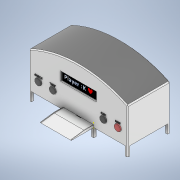
# Autodesk Inventor part: Twist Body
Saved by Autodesk Inventor 2021 (Build 250183000, 183)
## iProperties
Created: 2021-03-24
Part Number: Twist Body
Material: Generic
Document SubType Name: Modeling
Designer: calst
Density: 1 g/cm^3
Appearance: Smooth - White
Author: calst
Autodesk Inventor part; units mm, degrees
ref_plane "YZ Plane" through (0, 0, 0) normal (1, 0, 0) x (0, 1, 0)
ref_plane "XZ Plane" through (0, 0, 0) normal (0, 1, 0) x (-1, 0, 0)
sketch "Sketch1" plane through (0, 0, 0) normal (0, 1, 0) x (-1, 0, 0)
  line L0 (0, 0) -> (68.5, 0)
  line L1 (68.5, 0) -> (68.5, -94)
  line L2 (68.5, -94) -> (0, -94)
  line L3 (0, -94) -> (0, 0)
  dimension "d0" = 94
  dimension "d1" = 68.5
  constraints: 8 end point, 2 parallel, 1 horizontal, 1 perpendicular
  measures "d0" distance of L0.end L1.end
  measures "d1" distance of L1.end L2.end
extrude "Extrusion1" add sketch "Sketch1" along normal blind 4
sketch "Sketch2" plane through (0, 4, 0) normal (0, 1, 0) x (1, 0, 0)
  line L0 (0, 94) -> (-68.5, 94) projected
  line L1 (-68.5, 0) -> (0, 0) projected
  line L2 (-34.25, 0) -> (-39.25, 0)
  line L3 (-39.25, 0) -> (-39.25, 94)
  line L4 (-39.25, 94) -> (-29.25, 94)
  line L5 (-29.25, 94) -> (-29.25, 0)
  line L6 (-29.25, 0) -> (-34.25, 0)
  point P0 (-29.25, 0)
  dimension "d4" = 5
  dimension "d5" = 10
  constraints: 10 end point, 4 perpendicular, 1 midpoint, 1 point on line
  measures "d4" distance of L2.start L2.end
  measures "d5" distance of L3.end L4.end
extrude "Extrusion2" cut sketch "Sketch2" against normal blind 5
sketch "Sketch3" plane through (0, 4, 0) normal (0, 1, 0) x (1, 0, 0)
  line L0 (-39.25, 94) -> (-68.5, 94) projected
  line L1 (-68.5, 94) -> (-64.1699, 94)
  line L2 (-66, 89) -> (-68.5, 89)
  line L3 (-68.5, 89) -> (-68.5, 94)
  line L4 (-66, 89) -> (-66, 91.5)
  line L5 (-66, 91.5) -> (-64.1699, 91.5)
  line L6 (-64.1699, 94) -> (-68.5, 94)
  line L7 (-68.5, 94) -> (-68.5, 0) projected
  line L8 (-68.5, 89) -> (-68.5, 94)
  line L9 (0, 94) -> (-5, 94)
  line L10 (0, 94) -> (-29.25, 94) projected
  line L11 (-5, 91.5) -> (-2.5, 91.5)
  line L12 (-2.5, 91.5) -> (-2.5, 89)
  line L13 (0, 0) -> (0, 94) projected
  line L14 (0, 89) -> (0, 94)
  line L15 (-64.1699, 91.5) -> (-5, 91.5)
  line L16 (-64.1699, 94) -> (-5, 94)
  line L17 (0, 89) -> (0, 0)
  line L18 (0, 0) -> (-68.5, 0)
  line L19 (-68.5, 0) -> (-68.5, 89)
  line L20 (-66, 89) -> (-66, 2.5)
  line L21 (-68.5, 0) -> (-39.25, 0) projected
  line L22 (-66, 2.5) -> (-2.5, 2.5)
  line L23 (-2.5, 2.5) -> (-2.5, 89)
  dimension "d8" = 5
  dimension "d9" = 5
  dimension "d11" = 2.5
  dimension "d12" = 2.5
  dimension "d13" = 2.5
  dimension "d15" = 86.5
  constraints: 38 end point, 5 perpendicular, 4 collinear, 2 horizontal, 2 parallel, 1 point on line, 1 vertical
  measures "d8" distance of L5.end L2.end
  measures "d9" distance of L2.end L0.end
  measures "d11" distance of L9.end L11.start
  measures "d12" distance of L1.end L5.end
  measures "d13" distance of L2.start L4.end
  measures "d15" distance of L2.start L20.end
extrude "Extrusion3" add sketch "Sketch3" along normal blind 5
sketch "Sketch4" plane through (-29.25, 0, 0) normal (0, 0, 1) x (1, 0, 0)
  line L0 (-10, 4) -> (-36.75, 4) projected
  line L1 (26.75, 4) -> (0, 4) projected
  line L2 (-36.75, 4) -> (26.75, 4)
  line L3 (26.75, 4) -> (26.75, 5.1)
  line L4 (-36.75, 4) -> (-36.75, 5.1)
  line L5 (-36.75, 5.1) -> (26.75, 5.1)
  point P0 (29.25, 0)
  point P1 (-39.25, 9)
  dimension "d19" = 1.1
  dimension "d20" = 1.1
  constraints: 8 end point, 2 perpendicular, 1 collinear
  measures "d19" distance of L1.start L3.end
  measures "d20" distance of L0.end L4.end
extrude "Extrusion4" cut sketch "Sketch4" against normal blind 5
sketch "Sketch5" plane through (0, 9, 0) normal (0, 1, 0) x (1, 0, 0)
  line L0 (-66, 2.5) -> (-66, 91.5) projected
  line L1 (-68.5, 94) -> (-68.5, 0) projected
  line L2 (-66, 91.5) -> (-68.5, 91.5)
  line L3 (-68.5, 91.5) -> (-68.5, 94)
  line L4 (-68.5, 94) -> (-66, 94)
  line L5 (-66, 94) -> (-66, 91.5)
  line L6 (0, 0) -> (0, 94) projected
  line L7 (-2.5, 91.5) -> (-29.25, 91.5) projected
  line L8 (0, 94) -> (-2.5, 94)
  line L9 (-2.5, 94) -> (-2.5, 91.5)
  line L10 (-2.5, 91.5) -> (0, 91.5)
  line L11 (0, 91.5) -> (0, 94)
  line L12 (-68.5, 0.034) -> (-66, 0.034)
  line L13 (-66, 0.034) -> (-66, 2.534)
  line L14 (-66, 2.534) -> (-68.5, 2.534)
  line L15 (-68.5, 2.534) -> (-68.5, 0.034)
  line L16 (-2.5, 2.5) -> (-66, 2.5) projected
  line L17 (-68.5, 0) -> (0, 0) projected
  line L18 (-2.5, 2.5) -> (0, 2.5)
  line L19 (0, 2.5) -> (0, 0)
  line L20 (0, 0) -> (-2.5, 0)
  line L21 (-2.5, 0) -> (-2.5, 2.5)
  dimension "d23" = 2.5
  constraints: 32 end point, 8 parallel, 4 horizontal, 4 perpendicular, 2 point on line, 1 other
  measures "d23" distance of L12.end L13.end
extrude "Extrusion5" add sketch "Sketch5" along normal blind 30 contours L13 L12 L1 L14 L0 | L18 L6 L17 L21 | L2 L1 L4 L5 | L10 L9 L8 L6
sketch "Sketch6" plane through (0, 4, 0) normal (0, 1, 0) x (1, 0, 0)
  line L0 (-39.25, 94) -> (-68.5, 94) projected
  line L1 (-68.5, 94) -> (-66.2, 94)
  line L2 (-66.2, 94) -> (-66.2, 91.7)
  line L3 (-68.5, 91.5) -> (-66, 91.5) projected
  line L4 (0, 0) -> (0, 94) projected
  line L5 (0, 0) -> (-2.3, 0)
  line L6 (-29.25, 0) -> (0, 0) projected
  line L7 (-2.3, 0) -> (-2.3, 2.3)
  line L8 (-66.2, 91.7) -> (-2.3, 91.7)
  line L9 (-2.3, 91.7) -> (-2.3, 2.3)
  line L10 (-2.3, 2.3) -> (-66.2, 2.3)
  line L11 (-66.2, 2.3) -> (-66.2, 91.7)
  dimension "d26" = 2.3
  dimension "d27" = 2.3
  dimension "d28" = 2.3
  dimension "d29" = 2.3
  constraints: 16 end point, 3 perpendicular, 2 parallel, 2 point on line, 1 horizontal
  measures "d26" distance of L0.end L1.end
  measures "d27" distance of L1.end L2.end
  measures "d28" distance of L4.start L5.end
  measures "d29" distance of L5.end L7.end
extrude "Extrusion6" cut sketch "Sketch6" along normal blind 50
sketch "Sketch8" plane through (0, 0, 0) normal (1, 0, 0) x (0, 0, -1)
  line L0 (0, 4) -> (91.7, 4) projected
  line L1 (0, 4) -> (-20, 4)
  line L2 (-50, 0) -> (-20, 4)
  line L3 (0, 4) -> (0, 0) projected
  line L4 (-50, 0) -> (0, 0)
  dimension "d32" = 20
  constraints: 6 end point, 1 collinear, 1 horizontal
  measures "d32" distance of L0.start L1.end
extrude "Extrusion7" add sketch "Sketch8" against normal blind 68.5
sketch "Sketch10" plane through (0, 0, -94) normal (1, 0, 0) x (0, 0, -1)
  line L0 (-114, 4) -> (-94, 4) projected
  line L1 (-94, 5.1) -> (-91.7, 5.1) projected
  line L2 (-114, 5.1) -> (-94, 5.1)
  line L3 (-114, 4) -> (-144, 0) projected
  line L4 (-144, 0) -> (-144, 1.1)
  line L5 (-144, 1.1) -> (-114, 5.1)
  line L6 (-144, 0) -> (-114, 4)
  line L7 (-94, 4) -> (-94, 5.1)
  line L8 (-94, 4) -> (-91.7, 4) projected
  line L9 (-94, 4) -> (-114, 4)
  point P0 (-94, 0)
  dimension "d37" = 1.1
  constraints: 12 end point, 1 collinear, 1 perpendicular, 1 vertical
  measures "d37" distance of L3.end L4.end
extrude "Extrusion8" add sketch "Sketch10" against normal blind 1
sketch "Sketch11" plane through (-68.5, 4, 0) normal (-1, 0, 0) x (0, 0, 1)
  line L0 (50, -4) -> (20, 0) projected
  line L1 (50, -4) -> (50, -2.9) projected
  line L2 (50, -4) -> (50, -2.9)
  line L3 (20, 1.1) -> (0, 1.1) projected
  line L4 (50, -2.9) -> (20, 1.1)
  line L5 (20, 1.1) -> (0, 1.1)
  line L6 (0, 1.1) -> (0, 0) projected
  line L7 (0, 1.1) -> (0, 0)
  line L8 (20, 0) -> (0, 0) projected
  line L9 (0, 0) -> (20, 0)
  line L10 (50, -4) -> (-94, -4) projected
  line L11 (20, 0) -> (50, -4)
  point P0 (0, -4)
  constraints: 12 end point, 4 equal length, 1 perpendicular
extrude "Extrusion9" add sketch "Sketch11" against normal blind 1
sketch "Sketch15" plane through (-66.2, 4, -91.7) normal (0, 0, 1) x (1, 0, 0)
  line L0 (26.95, 0) -> (36.95, 0)
  line L1 (36.95, 0) -> (36.95, 1.1)
  line L2 (36.95, 1.1) -> (26.95, 1.1)
  line L3 (26.95, 1.1) -> (26.95, 0)
  point P0 (66.2, -4)
  dimension "d56" = 1.1
  constraints: 8 end point, 2 parallel, 1 horizontal, 1 perpendicular
  measures "d56" distance of L0.end L1.end
extrude "Extrusion13" cut sketch "Sketch15" against normal blind 94
sketch "Sketch17" plane through (0, 0, 0) normal (0, -1, 0) x (1, 0, 0)
  line L0 (-29.25, -81.7) -> (-24.25, -81.7)
  line L1 (-24.25, -81.7) -> (-24.25, -101.7)
  line L2 (-24.25, -101.7) -> (-29.25, -101.7)
  line L3 (-29.25, -101.7) -> (-29.25, -81.7)
  line L4 (-66, -2.3) -> (-2.5, -2.3) projected
  line L5 (-29.25, 0) -> (-39.25, 0) projected
  line L6 (-2.5, -2.3) -> (-66, -2.3) projected
  line L7 (-29.25, -2.3) -> (-29.25, -12.3)
  line L8 (-29.25, -91.7) -> (-29.25, 0) projected
  line L9 (-29.25, -12.3) -> (-24.25, -12.3)
  line L10 (-24.25, -12.3) -> (-24.25, 7.7)
  line L11 (-24.25, 7.7) -> (-29.25, 7.7)
  line L12 (-29.25, 7.7) -> (-29.25, -2.3)
  line L13 (-39.25, -2.3) -> (-39.25, -12.3)
  line L14 (-39.25, 0) -> (-39.25, -91.7) projected
  line L15 (-39.25, -12.3) -> (-44.25, -12.3)
  line L16 (-44.25, -12.3) -> (-44.25, 7.7)
  line L17 (-44.25, 7.7) -> (-39.25, 7.7)
  line L18 (-39.25, 7.7) -> (-39.25, -2.3)
  point P0 (0, 0)
  point P1 (-39.25, -81.7)
  dimension "d76" = 2.3
  dimension "d77" = 10
  dimension "d78" = 5
  dimension "d79" = 20
  constraints: 28 end point, 7 perpendicular, 6 point on line, 2 collinear, 1 horizontal
  measures "d76" distance between parallel lines of L4 L5
  measures "d77" distance of L7.start L7.end
  measures "d78" distance of L7.end L9.end
  measures "d79" distance of L9.end L10.end
extrude "Extrusion14" add sketch "Sketch17" along normal blind 20 contours L0 L1 L2 L3 | L13 L15 L16 L4 | L4 L16 L17 L18 L14 | L8 L12 L11 L10 L4 | L4 L10 L9 L7
fillet "Fillet1" radius 10 6 edges at (-26.75, -20, -81.7) (-26.75, -20, -101.7) (-26.75, -20, 7.7) (-26.75, -20, -12.3) (-41.75, -20, -12.3) (-41.75, -20, 7.7)
sketch "Sketch19" plane through (-24.25, 0, 7.7) normal (1, 0, 0) x (0, 0, -1)
  arc A0 (0, -10) -> (20, -10) centre (10, -10) ccw projected
  circle A1 centre (10, -10) radius 2.5
  arc A2 (89.4, -10) -> (109.4, -10) centre (99.4, -10) ccw projected
  circle A3 centre (99.4, -10) radius 2.5
  point P0 (7.7, 0)
  dimension "d80" = 5
  dimension "d81" = 5
  constraints: 2 centre point, 2 coincident
  measures "d80" diameter of A1
  measures "d81" diameter of A3
extrude "Extrusion16" cut sketch "Sketch19" against normal blind 30
sketch "Sketch21" plane through (0, 0, 0) normal (0, -1, 0) x (1, 0, 0)
  line L0 (-68.5, -94) -> (-63.5, -94)
  line L1 (-63.5, -94) -> (-63.5, -89)
  line L2 (-63.5, -89) -> (-68.5, -89)
  line L3 (-68.5, -89) -> (-68.5, -94)
  line L4 (-67.5, 50) -> (-68.5, 50) projected
  line L5 (0, 50) -> (-1, 50) projected
  line L6 (0, -94) -> (-2.5, -94) projected
  line L7 (0, -94) -> (-5, -94)
  line L8 (-5, -94) -> (-5, -89)
  line L9 (-5, -89) -> (0, -89)
  line L10 (0, -89) -> (0, -94)
  dimension "d84" = 5
  dimension "d85" = 5
  constraints: 16 end point, 4 parallel, 2 horizontal, 2 perpendicular
  measures "d84" distance of L0.end L1.end
  measures "d85" distance of L1.end L2.end
extrude "Extrusion17" add sketch "Sketch21" along normal blind 20
sketch "Sketch23" plane through (0, 9, -91.5) normal (1, 0, 0) x (0, 0, -1)
  point P0 (-91.5, -9)
sketch "Sketch24" plane through (0, 0, 0) normal (0, -1, 0) x (1, 0, 0)
  line L0 (0, 0) -> (-5, 0)
  line L1 (-5, 0) -> (-5, -5)
  line L2 (-5, -5) -> (0, -5)
  line L3 (0, -5) -> (0, 0)
  line L4 (-68.5, -0.034) -> (-68.5, 0) projected
  line L5 (-68.5, 0) -> (-63.5, 0)
  line L6 (-63.5, 0) -> (-63.5, -5)
  line L7 (-63.5, -5) -> (-68.5, -5)
  line L8 (-68.5, -5) -> (-68.5, 0)
  dimension "d94" = 5
  dimension "d95" = 5
  dimension "d96" = 5
  constraints: 16 end point, 4 parallel, 2 horizontal, 2 perpendicular
  measures "d94" distance of L2.end L1.end
  measures "d95" distance of L0.end L1.end
  measures "d96" distance of L6.end L7.end
extrude "Extrusion18" add sketch "Sketch24" along normal blind 20
sketch "Sketch25" plane through (0, 9, -91.5) normal (1, 0, 0) x (0, 0, -1)
  line L0 (-91.466, 0) -> (-91.5, 0) projected
  line L1 (-9.8, -9) -> (2.5, -9) projected
  line L2 (-91.5, 0) -> (2.5, 0)
  line L3 (2.5, 0) -> (2.5, -9)
  line L4 (2.5, -9) -> (-91.5, -9)
  line L5 (-91.5, -9) -> (-91.5, 0)
  point P0 (-91.5, -9)
  constraints: 8 end point, 2 parallel, 1 horizontal, 1 perpendicular
extrude "Extrusion19" add sketch "Sketch25" along normal blind 75
sketch "Sketch26" plane through (-68.5, 9, -0.034) normal (-1, 0, 0) x (0, 0, 1)
  line L0 (0.034, -9) -> (0.034, -29) projected
  line L1 (-93.966, 0) -> (0.034, 0)
  line L2 (0.034, 0) -> (0.034, -9)
  line L3 (0.034, -9) -> (-93.966, -9)
  line L4 (-93.966, -9) -> (-93.966, 0)
  constraints: 8 end point, 2 parallel, 1 horizontal, 1 perpendicular
extrude "Extrusion20" add sketch "Sketch26" along normal blind 75
sketch "Sketch28" plane through (0, 0, 0) normal (0, -1, 0) x (1, 0, 0)
  line L0 (-68.5, -94) -> (-143.5, -94) projected
  line L1 (-143.5, -94) -> (-138.5, -94)
  line L2 (-138.5, -94) -> (-138.5, -89)
  line L3 (-138.5, -89) -> (-143.5, -89)
  line L4 (-143.5, -89) -> (-143.5, -94)
  line L5 (-143.5, -94) -> (-143.5, 0) projected
  line L6 (-143.5, 0) -> (-138.5, 0)
  line L7 (-138.5, 0) -> (-138.5, -5)
  line L8 (-138.5, -5) -> (-143.5, -5)
  line L9 (-143.5, -5) -> (-143.5, 0)
  line L10 (0, -94) -> (75, -94) projected
  line L11 (75, -94) -> (70, -94)
  line L12 (70, -94) -> (70, -89)
  line L13 (70, -89) -> (75, -89)
  line L14 (75, -89) -> (75, -94)
  line L15 (75, -94) -> (75, 0) projected
  line L16 (75, 0) -> (70, 0)
  line L17 (70, 0) -> (70, -5)
  line L18 (70, -5) -> (75, -5)
  line L19 (75, -5) -> (75, 0)
  point P0 (0, 0)
  dimension "d103" = 5
  dimension "d104" = 5
  dimension "d105" = 5
  dimension "d106" = 5
  dimension "d107" = 5
  dimension "d108" = 5
  constraints: 32 end point, 8 parallel, 4 horizontal, 4 perpendicular, 2 point on line
  measures "d103" distance of L3.end L2.end
  measures "d104" distance of L12.end L13.end
  measures "d105" distance of L18.end L17.end
  measures "d106" distance of L6.end L7.end
  measures "d107" distance of L1.end L2.end
  measures "d108" distance of L16.end L17.end
extrude "Extrusion21" add sketch "Sketch28" along normal blind 20
sketch "Sketch29" plane through (0, 9, 0) normal (0, 1, 0) x (1, 0, 0)
  point P0 (0, 0)
sketch "Sketch30" plane through (0, 9, 0) normal (0, 1, 0) x (1, 0, 0)
  line L0 (2.7, 89) -> (70, 89)
  line L1 (70, 89) -> (70, 5)
  line L2 (70, 5) -> (2.7, 5)
  line L3 (2.7, 5) -> (2.7, 89)
  line L4 (-138.5, 94) -> (-138.5, 89) projected
  line L5 (-138.5, 89) -> (-71.2, 89)
  line L6 (-71.2, 89) -> (-71.2, 5)
  line L7 (-71.2, 5) -> (-138.5, 5)
  line L8 (-138.5, 5) -> (-138.5, 89)
  line L9 (-2.5, 0) -> (-143.5, 0) projected
  line L10 (-66.2, 2.534) -> (-66.2, 91.5) projected
  line L11 (0, 94) -> (75, 94) projected
  line L12 (75, 94) -> (75, 0) projected
  line L13 (-2.3, 91.5) -> (-2.3, 2.5) projected
  point P0 (0, 0)
  dimension "d111" = 5
  dimension "d112" = 5
  dimension "d113" = 5
  dimension "d114" = 5
  dimension "d115" = 5
  constraints: 16 end point, 4 parallel, 2 horizontal, 2 perpendicular, 1 point on line
  measures "d111" distance between parallel lines of L9 L7
  measures "d112" distance between parallel lines of L10 L6
  measures "d113" distance between parallel lines of L11 L0
  measures "d114" distance between parallel lines of L12 L1
  measures "d115" distance between parallel lines of L13 L3
extrude "Extrusion22" cut sketch "Sketch30" against normal blind 5
sketch "Sketch32" plane through (0, 9, 0) normal (0, 1, 0) x (1, 0, 0)
  line L0 (-68.5, 94) -> (-143.5, 94) projected
  line L1 (75, 5) -> (75, 0) projected
  line L2 (-143.5, 94) -> (75, 94)
  line L3 (75, 94) -> (75, 0)
  line L4 (75, 0) -> (-143.5, 0)
  line L5 (-143.5, 0) -> (-143.5, 94)
  line L6 (-71.2, 89) -> (-71.2, 5) projected
  line L7 (-138.5, 89) -> (-71.2, 89)
  line L8 (-71.2, 89) -> (-71.2, 5)
  line L9 (-71.2, 5) -> (-138.5, 5)
  line L10 (-138.5, 5) -> (-138.5, 89)
  line L11 (70, 89) -> (70, 5) projected
  line L12 (2.7, 89) -> (70, 89)
  line L13 (70, 89) -> (70, 5)
  line L14 (70, 5) -> (2.7, 5)
  line L15 (2.7, 5) -> (2.7, 89)
  line L16 (-66.2, 2.534) -> (-66.2, 91.5) projected
  line L17 (-2.5, 91.7) -> (-2.3, 91.7) projected
  line L18 (-66.2, 2.534) -> (-2.3, 2.534)
  line L19 (-2.3, 2.534) -> (-2.3, 91.7)
  line L20 (-2.3, 91.7) -> (-66.2, 91.7)
  line L21 (-66.2, 91.7) -> (-66.2, 2.534)
  point P0 (0, 0)
  constraints: 32 end point, 8 parallel, 4 horizontal, 4 perpendicular
extrude "Extrusion23" add sketch "Sketch32" along normal blind 30
chamfer "Chamfer1" distance 2 angle 45 2 edges at (-143.5, 9.5, 0) (75, 9.5, 0)
sketch "Sketch34" plane through (-138.5, 39, -5) normal (1, 0, 0) x (0, 0, -1)
  line L0 (-3, 0) -> (-3, -59) projected
  line L1 (0, 0) -> (84, 0) projected
  line L2 (-3, 0) -> (84, 0)
  line L3 (84, 0) -> (84, -2.5)
  line L4 (84, 0) -> (84, -35) projected
  line L5 (84, -2.5) -> (-3, -2.5)
  line L6 (-3, -2.5) -> (-3, 0)
  point P0 (-5, -39)
  point P1 (84, -15)
  point P2 (-3, -2.5)
  dimension "d129" = 2.5
  constraints: 8 end point, 2 perpendicular, 1 collinear, 1 point on line
  measures "d129" distance of L1.end L3.end
extrude "Extrusion25" add sketch "Sketch34" along normal blind 68
sketch "Sketch35" plane through (2.7, 39, -5) normal (1, 0, 0) x (0, 0, -1)
  line L0 (0, -2.5) -> (0, -35) projected
  line L1 (0, 0) -> (0, -2.5)
  line L2 (84, -2.5) -> (84, -35) projected
  line L3 (0, -2.5) -> (84, -2.5)
  line L4 (84, -2.5) -> (84, 0)
  line L5 (84, 0) -> (0, 0)
  point P0 (-5, -39)
  point P1 (0, -15)
  point P2 (84, -15)
  constraints: 8 end point, 2 perpendicular, 1 parallel, 1 vertical
extrude "Extrusion26" add sketch "Sketch35" along normal blind 68
sketch "Sketch36" plane through (0, 39, 0) normal (0, 1, 0) x (1, 0, 0)
  line L0 (-66.2, 2.534) -> (-66.2, 91.7) projected
  line L1 (-143.5, 94) -> (-143.5, 2) projected
  line L2 (-68.5, 0) -> (-138.5, 0) projected
  line L3 (-92.35, 42.117) -> (-117.35, 42.117)
  line L4 (-117.35, 42.117) -> (-117.35, 52.117)
  line L5 (-117.35, 52.117) -> (-92.35, 52.117)
  line L6 (-92.35, 52.117) -> (-92.35, 42.117)
  line L7 (-92.35, 42.117) -> (-117.35, 52.117) construction
  line L8 (-117.35, 42.117) -> (-92.35, 52.117) construction
  line L9 (48.85, 42.117) -> (23.85, 42.117)
  line L10 (23.85, 42.117) -> (23.85, 52.117)
  line L11 (23.85, 52.117) -> (48.85, 52.117)
  line L12 (48.85, 52.117) -> (48.85, 42.117)
  line L13 (48.85, 42.117) -> (23.85, 52.117) construction
  line L14 (23.85, 42.117) -> (48.85, 52.117) construction
  line L15 (-141.5, 0) -> (73, 0) projected
  line L16 (75, 2) -> (75, 94) projected
  line L17 (-2.3, 91.7) -> (-2.3, 2.534) projected
  point P0 (0, 0)
  point P1 (36.35, 47.117)
  dimension "d134" = 25
  dimension "d135" = 10
  dimension "d136" = 42.117
  dimension "d137" = 26.15
  dimension "d138" = 25
  dimension "d139" = 42.117
  dimension "d140" = 26.15
  dimension "d185" = 26.15
  dimension "d186" = 26.15
  constraints: 24 end point, 4 parallel, 2 horizontal, 2 midpoint, 2 perpendicular
  measures "d134" distance of L4.end L5.end
  measures "d135" distance of L3.end L4.end
  measures "d136" distance between parallel lines of L2 L3
  measures "d137" distance between parallel lines of L1 L4
  measures "d138" distance of L10.end L11.end
  measures "d139" distance between parallel lines of L15 L9
  measures "d140" distance between parallel lines of L16 L12
  measures "d185" distance between parallel lines of L17 L10
  measures "d186" distance between parallel lines of L0 L6
extrude "Extrusion27" cut sketch "Sketch36" against normal blind 2.5
sketch "Sketch37" plane through (-138.5, 36.5, -89) normal (0, -1, 0) x (1, 0, 0)
  line L0 (21.15, 46.883) -> (46.15, 46.883) projected
  line L1 (21.15, 46.883) -> (41.15, 46.883)
  line L2 (41.15, 46.883) -> (41.15, 51.883)
  line L3 (41.15, 51.883) -> (21.15, 51.883)
  line L4 (21.15, 51.883) -> (21.15, 46.883)
  line L5 (162.35, 46.883) -> (182.35, 46.883)
  line L6 (182.35, 46.883) -> (182.35, 51.883)
  line L7 (182.35, 51.883) -> (162.35, 51.883)
  line L8 (162.35, 51.883) -> (162.35, 46.883)
  point P0 (138.5, 89)
  point P1 (41.15, 46.883)
  dimension "d143" = 5
  dimension "d144" = 20
  constraints: 16 end point, 4 parallel, 2 horizontal, 2 perpendicular
  measures "d143" distance of L3.end L0.start
  measures "d144" distance of L7.end L6.end
extrude "Extrusion28" add sketch "Sketch37" along normal blind 20
fillet "Fillet2" radius 10 4 edges at (43.85, 16.5, -39.617) (23.85, 16.5, -39.617) (-97.35, 16.5, -39.617) (-117.35, 16.5, -39.617)
sketch "Sketch38" plane through (23.85, 36.5, -37.117) normal (0, 0, 1) x (1, 0, 0)
  arc A0 (0, -10) -> (20, -10) centre (10, -10) ccw projected
  circle A1 centre (10, -10) radius 2.5
  arc A2 (-141.2, -10) -> (-121.2, -10) centre (-131.2, -10) ccw projected
  circle A3 centre (-131.2, -10) radius 2.5
  point P0 (-23.85, -36.5)
  dimension "d148" = 5
  dimension "d149" = 5
  constraints: 2 centre point, 2 coincident
  measures "d148" diameter of A1
  measures "d149" diameter of A3
extrude "Extrusion29" cut sketch "Sketch38" against normal blind 5
sketch "Sketch39" plane through (0, 39, 0) normal (0, 1, 0) x (1, 0, 0)
  line L0 (-143.5, 94) -> (-143.5, 2) projected
  line L1 (75, 94) -> (-143.5, 94) projected
  line L2 (-141.5, 0) -> (73, 0) projected
  line L3 (75, 2) -> (75, 94) projected
  line L4 (75, 2) -> (73, 0) projected
  line L5 (-141.5, 0) -> (-143.5, 2) projected
  line L6 (-66.2, 91.7) -> (-2.3, 91.7) projected
  line L7 (-2.3, 2.534) -> (-66.2, 2.534) projected
  line L8 (-39.25, 91.7) -> (-66.2, 91.7) projected
  line L9 (-66.2, 91.7) -> (-141.2, 91.7)
  line L10 (-2.3, 91.7) -> (72.7, 91.7)
  line L11 (-66, 0) -> (-66, 2.3) projected
  line L12 (-66, 2.3) -> (-141.2, 2.3)
  line L13 (-141.2, 2.3) -> (-141.2, 91.7)
  line L14 (-66, 2.3) -> (-2.5, 2.3) projected
  line L15 (-66, 2.3) -> (72.7, 2.3)
  line L16 (72.7, 91.7) -> (72.7, 2.3)
  line L17 (-66.2, 91.7) -> (-2.3, 91.7)
  line L18 (-2.5, 2.3) -> (-66, 2.3)
  line L19 (-143.5, 94) -> (75, 94)
  line L20 (75, 2) -> (75, 94)
  line L21 (73, 0) -> (75, 2)
  line L22 (75, 2) -> (73, 0)
  line L23 (73, 0) -> (70, 0) projected
  line L24 (-141.5, 0) -> (73, 0)
  line L25 (-143.5, 89) -> (-143.5, 94) projected
  line L26 (-143.5, 2) -> (-143.5, 94)
  line L27 (-141.5, 0) -> (-143.5, 2)
  point P0 (0, 0)
  dimension "d153" = 2.3
  dimension "d154" = 2.3
  dimension "d155" = 2.3
  constraints: 30 end point, 4 horizontal, 2 collinear, 2 perpendicular, 2 vertical, 1 parallel, 1 point on line
  measures "d153" distance between parallel lines of L1 L9
  measures "d154" distance from line of L0 L9.end
  measures "d155" distance from line of L3 L10.end
extrude "Extrusion30" add sketch "Sketch39" along normal blind 40
sketch "Sketch40" plane through (-29.25, 5.1, -94) normal (0, 0, -1) x (-1, 0, 0)
  line L0 (114.25, 73.9) -> (112.25, 73.9) projected
  arc A0 (114.25, 73.9) -> (-104.25, 73.9) centre (5, -150.9654) ccw
  line L1 (-104.25, 73.9) -> (114.25, 73.9)
  line L2 (-102.25, 73.9) -> (-102.25, -25.1) projected
  point P0 (-29.25, -5.1)
  dimension "d158" = 250
  constraints: 2 end point, 2 point on circle, 1 centre point, 1 perpendicular
  measures "d158" radius of A0
extrude "Extrusion31" add sketch "Sketch40" against normal blind 94
chamfer "Chamfer2" distance 2 angle 45 1 edges at (-34.25, 104.1346, 0)
chamfer "Chamfer3" distance 2 angle 45 5 edges at (-143.5, 29.5, -94) (75, 29.5, -94) (-34.25, 104.1346, -94) (-143.5, 79, -48) (75, 79, -48)
sketch "Sketch41" plane through (-66, 5.1, 0) normal (0, 0, 1) x (1, 0, 0)
  arc A0 (139, 72.6446) -> (-75.5, 72.6446) centre (31.75, -150.9654) ccw projected
  line L0 (31.75, 47.0346) -> (71.75, 47.0346)
  line L1 (71.75, 47.0346) -> (71.75, 67.0346)
  line L2 (31.75, 47.0346) -> (-8.25, 47.0346)
  line L3 (-8.25, 47.0346) -> (-8.25, 67.0346)
  line L4 (-8.25, 67.0346) -> (71.75, 67.0346)
  point P0 (66, -5.1)
  dimension "d170" = 40
  dimension "d171" = 20
  dimension "d172" = 40
  dimension "d173" = 20
  constraints: 10 end point, 2 perpendicular, 1 horizontal
  measures "d170" distance of L0.start L0.end
  measures "d171" distance of L0.end L1.end
  measures "d172" distance of L0.start L2.end
  measures "d173" distance of L2.end L3.end
extrude "Extrusion32" cut sketch "Sketch41" against normal blind 2.2
ref_plane "Work Plane1" through (-66, 5.1, 28.05) normal (0, 0, 1) x (1, 0, 0)
sketch "Sketch43" plane through (-66, 5.1, 28.05) normal (0, 0, 1) x (1, 0, 0)
  line L0 (-6.2731, 67.1185) -> (70.6599, 67.1185) construction
  line L1 (70.6599, 67.1185) -> (70.6599, 47.1186) construction
  line L2 (70.6599, 47.1186) -> (-6.2731, 47.1186) construction
  line L3 (-6.2731, 47.1186) -> (-6.2731, 67.1185) construction
  point P0 (66, -5.1)
  constraints: 2 other
decal "Decal1"
sketch "Sketch44" plane through (-66, 5.1, 0) normal (0, 0, 1) x (1, 0, 0)
  line L0 (71.75, 47.0346) -> (-8.25, 47.0346) projected
  line L1 (31.75, 47.0346) -> (31.75, 22.0346)
  line L2 (-72.5, -1.1) -> (-72.5, 31.4) projected
  line L3 (-8.25, 22.0346) -> (-8.25, 15.15)
  line L4 (-5.2, 31.4) -> (-5.2, -1.1) projected
  circle A0 centre (-56.4375, 22.0346) radius 7.5
  circle A1 centre (-24.3125, 22.0346) radius 7.5
  line L5 (136, -1.1) -> (136, 31.4) projected
  circle A2 centre (119.9375, 22.0346) radius 7.5
  circle A3 centre (87.8125, 22.0346) radius 7.5
  point P0 (66, -5.1)
  dimension "d187" = 25
  dimension "d189" = 15
  dimension "d190" = 15
  dimension "d191" = 15
  dimension "d192" = 15
  constraints: 4 centre point, 4 end point, 2 vertical, 1 midpoint
  measures "d187" distance of L1.start L1.end
  measures "d189" diameter of A0
  measures "d190" diameter of A1
  measures "d191" diameter of A2
  measures "d192" diameter of A3
extrude "Extrusion33" cut sketch "Sketch44" against normal blind 2.2
sketch "Sketch45" plane through (-90.3125, 27.1346, -2.2) normal (0, 0, 1) x (1, 0, 0)
  circle A0 centre (-32.125, 0) radius 7.5 projected
  circle A1 centre (-32.125, 0) radius 7
  circle A2 centre (0, 0) radius 7.5 projected
  circle A3 centre (0, 0) radius 7
  circle A4 centre (112.125, 0) radius 7.5 projected
  circle A5 centre (112.125, 0) radius 7
  circle A6 centre (144.25, 0) radius 7.5 projected
  circle A7 centre (144.25, 0) radius 7
  point P0 (90.3125, -27.1346)
  dimension "d195" = 14
  dimension "d196" = 14
  dimension "d197" = 14
  dimension "d198" = 14
  constraints: 4 centre point, 4 coincident
  measures "d195" diameter of A1
  measures "d196" diameter of A3
  measures "d197" diameter of A5
  measures "d198" diameter of A7
extrude "Extrusion34" add sketch "Sketch45" along normal blind 4 contours A1 | A3 | A5 | A7
sketch "Sketch46" plane through (-66, 5.1, 0) normal (0, 0, 1) x (1, 0, 0)
  line L0 (-64.6481, 33.6434) -> (-37.5549, 33.6434) construction
  line L1 (-37.5549, 33.6434) -> (-37.5549, 35.8702) construction
  line L2 (-37.5549, 35.8702) -> (-64.6481, 35.8702) construction
  line L3 (-64.6481, 35.8702) -> (-64.6481, 33.6434) construction
  line L4 (-31.0201, 33.5651) -> (-3.9269, 33.5651) construction
  line L5 (-3.9269, 33.5651) -> (-3.9269, 35.792) construction
  line L6 (-3.9269, 35.792) -> (-31.0201, 35.792) construction
  line L7 (-31.0201, 35.792) -> (-31.0201, 33.5651) construction
  line L8 (113.8778, 33.6168) -> (113.8778, 33.6618) construction
  line L9 (113.8778, 33.6618) -> (140.971, 33.6618) construction
  line L10 (140.971, 33.6618) -> (140.971, 33.6168) construction
  line L11 (140.971, 33.6168) -> (113.8778, 33.6168) construction
  line L12 (82.1971, 35.8299) -> (82.1971, 33.6031) construction
  line L13 (82.1971, 33.6031) -> (109.2903, 33.6031) construction
  line L14 (109.2903, 33.6031) -> (109.2903, 35.8299) construction
  line L15 (109.2903, 35.8299) -> (82.1971, 35.8299) construction
  spline S0 degree 2 poles (-63.4897, 30.4867) (-63.8206, 30.4867) (-64.285, 30.625) (-64.49, 30.7238) knots 0 0 0 1 2 2 2
  line L16 (-64.49, 30.7238) -> (-64.49, 31.2326)
  line L17 (-64.49, 31.2326) -> (-64.4604, 31.2326)
  spline S1 degree 2 poles (-64.4604, 31.2326) (-64.2603, 31.0449) (-63.754, 30.8374) (-63.5193, 30.8374) knots 0 0 0 1 2 2 2
  spline S2 degree 2 poles (-63.5193, 30.8374) (-63.1834, 30.8374) (-62.8401, 31.1165) (-62.8401, 31.3462) knots 0 0 0 1 2 2 2
  spline S3 degree 2 poles (-62.8401, 31.3462) (-62.8401, 31.529) (-63.0204, 31.7563) (-63.2155, 31.8131) knots 0 0 0 1 2 2 2
  spline S4 degree 2 poles (-63.2155, 31.8131) (-63.3563, 31.8526) (-63.5909, 31.9069) (-63.7663, 31.9514) knots 0 0 0 1 2 2 2
  spline S5 degree 2 poles (-63.7663, 31.9514) (-63.9244, 31.9934) (-64.1739, 32.1194) (-64.2702, 32.2206) knots 0 0 0 1 2 2 2
  spline S6 degree 2 poles (-64.2702, 32.2206) (-64.3641, 32.3219) (-64.4678, 32.5936) (-64.4678, 32.7714) knots 0 0 0 1 2 2 2
  spline S7 degree 2 poles (-64.4678, 32.7714) (-64.4678, 33.1419) (-63.8898, 33.6434) (-63.4427, 33.6434) knots 0 0 0 1 2 2 2
  spline S8 degree 2 poles (-63.4427, 33.6434) (-63.1859, 33.6434) (-62.7314, 33.5421) (-62.5362, 33.4458) knots 0 0 0 1 2 2 2
  line L18 (-62.5362, 33.4458) -> (-62.5362, 32.9616)
  line L19 (-62.5362, 32.9616) -> (-62.5659, 32.9616)
  spline S9 degree 2 poles (-62.5659, 32.9616) (-62.7116, 33.095) (-63.1661, 33.2926) (-63.4156, 33.2926) knots 0 0 0 1 2 2 2
  spline S10 degree 2 poles (-63.4156, 33.2926) (-63.6971, 33.2926) (-64.0454, 33.0283) (-64.0454, 32.8134) knots 0 0 0 1 2 2 2
  spline S11 degree 2 poles (-64.0454, 32.8134) (-64.0454, 32.6208) (-63.8404, 32.3911) (-63.6477, 32.3392) knots 0 0 0 1 2 2 2
  spline S12 degree 2 poles (-63.6477, 32.3392) (-63.5193, 32.3046) (-63.1463, 32.2157) (-63.0228, 32.1786) knots 0 0 0 1 2 2 2
  spline S13 degree 2 poles (-63.0228, 32.1786) (-62.7091, 32.0823) (-62.4177, 31.6945) (-62.4177, 31.4105) knots 0 0 0 1 2 2 2
  spline S14 degree 2 poles (-62.4177, 31.4105) (-62.4177, 31.2302) (-62.5634, 30.8844) (-62.6943, 30.7633) knots 0 0 0 1 2 2 2
  spline S15 degree 2 poles (-62.6943, 30.7633) (-62.8401, 30.6299) (-63.2106, 30.4867) (-63.4897, 30.4867) knots 0 0 0 1 2 2 2
  line L20 (-59.7921, 30.541) -> (-60.1971, 30.541)
  line L21 (-60.1971, 30.541) -> (-60.1971, 32.0329)
  line L22 (-60.1971, 32.0329) -> (-61.6001, 32.0329)
  line L23 (-61.6001, 32.0329) -> (-61.6001, 30.541)
  line L24 (-61.6001, 30.541) -> (-62.0052, 30.541)
  line L25 (-62.0052, 30.541) -> (-62.0052, 33.589)
  line L26 (-62.0052, 33.589) -> (-61.6001, 33.589)
  line L27 (-61.6001, 33.589) -> (-61.6001, 32.3935)
  line L28 (-61.6001, 32.3935) -> (-60.1971, 32.3935)
  line L29 (-60.1971, 32.3935) -> (-60.1971, 33.589)
  line L30 (-60.1971, 33.589) -> (-59.7921, 33.589)
  line L31 (-59.7921, 33.589) -> (-59.7921, 30.541)
  spline S16 degree 2 poles (-58.11, 30.4768) (-58.3792, 30.4768) (-58.7793, 30.6176) (-58.9201, 30.7584) knots 0 0 0 1 2 2 2
  spline S17 degree 2 poles (-58.9201, 30.7584) (-59.0807, 30.9165) (-59.2116, 31.3611) (-59.2116, 31.6871) knots 0 0 0 1 2 2 2
  line L32 (-59.2116, 31.6871) -> (-59.2116, 33.589)
  line L33 (-59.2116, 33.589) -> (-58.8065, 33.589)
  line L34 (-58.8065, 33.589) -> (-58.8065, 31.6871)
  spline S18 degree 2 poles (-58.8065, 31.6871) (-58.8065, 31.4747) (-58.7522, 31.1882) (-58.6756, 31.0721) knots 0 0 0 1 2 2 2
  spline S19 degree 2 poles (-58.6756, 31.0721) (-58.5941, 30.9486) (-58.3125, 30.8226) (-58.11, 30.8226) knots 0 0 0 1 2 2 2
  spline S20 degree 2 poles (-58.11, 30.8226) (-57.9198, 30.8226) (-57.6234, 30.9486) (-57.5419, 31.0721) knots 0 0 0 1 2 2 2
  spline S21 degree 2 poles (-57.5419, 31.0721) (-57.4653, 31.1882) (-57.411, 31.4722) (-57.411, 31.6772) knots 0 0 0 1 2 2 2
  line L35 (-57.411, 31.6772) -> (-57.411, 33.589)
  line L36 (-57.411, 33.589) -> (-57.0059, 33.589)
  line L37 (-57.0059, 33.589) -> (-57.0059, 31.6871)
  spline S22 degree 2 poles (-57.0059, 31.6871) (-57.0059, 31.3685) (-57.1343, 30.914) (-57.2973, 30.7584) knots 0 0 0 1 2 2 2
  spline S23 degree 2 poles (-57.2973, 30.7584) (-57.4431, 30.6151) (-57.8284, 30.4768) (-58.11, 30.4768) knots 0 0 0 1 2 2 2
  line L38 (-54.6025, 33.2284) -> (-56.0203, 33.2284)
  line L39 (-56.0203, 33.2284) -> (-56.0203, 32.3688)
  line L40 (-56.0203, 32.3688) -> (-54.6618, 32.3688)
  line L41 (-54.6618, 32.3688) -> (-54.6618, 32.0082)
  line L42 (-54.6618, 32.0082) -> (-56.0203, 32.0082)
  line L43 (-56.0203, 32.0082) -> (-56.0203, 30.541)
  line L44 (-56.0203, 30.541) -> (-56.4254, 30.541)
  line L45 (-56.4254, 30.541) -> (-56.4254, 33.589)
  line L46 (-56.4254, 33.589) -> (-54.6025, 33.589)
  line L47 (-54.6025, 33.589) -> (-54.6025, 33.2284)
  line L48 (-52.4166, 33.2284) -> (-53.8344, 33.2284)
  line L49 (-53.8344, 33.2284) -> (-53.8344, 32.3688)
  line L50 (-53.8344, 32.3688) -> (-52.4759, 32.3688)
  line L51 (-52.4759, 32.3688) -> (-52.4759, 32.0082)
  line L52 (-52.4759, 32.0082) -> (-53.8344, 32.0082)
  line L53 (-53.8344, 32.0082) -> (-53.8344, 30.541)
  line L54 (-53.8344, 30.541) -> (-54.2395, 30.541)
  line L55 (-54.2395, 30.541) -> (-54.2395, 33.589)
  line L56 (-54.2395, 33.589) -> (-52.4166, 33.589)
  line L57 (-52.4166, 33.589) -> (-52.4166, 33.2284)
  line L58 (-50.2874, 30.541) -> (-52.0535, 30.541)
  line L59 (-52.0535, 30.541) -> (-52.0535, 33.589)
  line L60 (-52.0535, 33.589) -> (-51.6484, 33.589)
  line L61 (-51.6484, 33.589) -> (-51.6484, 30.9016)
  line L62 (-51.6484, 30.9016) -> (-50.2874, 30.9016)
  line L63 (-50.2874, 30.9016) -> (-50.2874, 30.541)
  line L64 (-49.9688, 30.541) -> (-49.9688, 33.589)
  line L65 (-49.9688, 33.589) -> (-48.0619, 33.589)
  line L66 (-48.0619, 33.589) -> (-48.0619, 33.2284)
  line L67 (-48.0619, 33.2284) -> (-49.5637, 33.2284)
  line L68 (-49.5637, 33.2284) -> (-49.5637, 32.3935)
  line L69 (-49.5637, 32.3935) -> (-48.1632, 32.3935)
  line L70 (-48.1632, 32.3935) -> (-48.1632, 32.0329)
  line L71 (-48.1632, 32.0329) -> (-49.5637, 32.0329)
  line L72 (-49.5637, 32.0329) -> (-49.5637, 30.9016)
  line L73 (-49.5637, 30.9016) -> (-48.0619, 30.9016)
  line L74 (-48.0619, 30.9016) -> (-48.0619, 30.541)
  line L75 (-48.0619, 30.541) -> (-49.9688, 30.541)
  line L76 (-30, 30.4628) -> (-30, 33.1502)
  line L77 (-30, 33.1502) -> (-31.0225, 33.1502)
  line L78 (-31.0225, 33.1502) -> (-31.0225, 33.5108)
  line L79 (-31.0225, 33.5108) -> (-28.5723, 33.5108)
  line L80 (-28.5723, 33.5108) -> (-28.5723, 33.1502)
  line L81 (-28.5723, 33.1502) -> (-29.5949, 33.1502)
  line L82 (-29.5949, 33.1502) -> (-29.5949, 30.4628)
  line L83 (-29.5949, 30.4628) -> (-30, 30.4628)
  line L84 (-24.8475, 33.5108) -> (-25.6132, 30.4628)
  line L85 (-25.6132, 30.4628) -> (-26.0677, 30.4628)
  line L86 (-26.0677, 30.4628) -> (-26.6877, 32.9921)
  line L87 (-26.6877, 32.9921) -> (-27.2903, 30.4628)
  line L88 (-27.2903, 30.4628) -> (-27.7399, 30.4628)
  line L89 (-27.7399, 30.4628) -> (-28.5179, 33.5108)
  line L90 (-28.5179, 33.5108) -> (-28.1005, 33.5108)
  line L91 (-28.1005, 33.5108) -> (-27.4879, 30.984)
  line L92 (-27.4879, 30.984) -> (-26.8803, 33.5108)
  line L93 (-26.8803, 33.5108) -> (-26.4678, 33.5108)
  line L94 (-26.4678, 33.5108) -> (-25.8553, 30.9543)
  line L95 (-25.8553, 30.9543) -> (-25.2452, 33.5108)
  line L96 (-25.2452, 33.5108) -> (-24.8475, 33.5108)
  line L97 (-23.4223, 30.4628) -> (-24.603, 30.4628)
  line L98 (-24.603, 30.4628) -> (-24.603, 30.774)
  line L99 (-24.603, 30.774) -> (-24.2152, 30.774)
  line L100 (-24.2152, 30.774) -> (-24.2152, 33.1996)
  line L101 (-24.2152, 33.1996) -> (-24.603, 33.1996)
  line L102 (-24.603, 33.1996) -> (-24.603, 33.5108)
  line L103 (-24.603, 33.5108) -> (-23.4223, 33.5108)
  line L104 (-23.4223, 33.5108) -> (-23.4223, 33.1996)
  line L105 (-23.4223, 33.1996) -> (-23.8101, 33.1996)
  line L106 (-23.8101, 33.1996) -> (-23.8101, 30.774)
  line L107 (-23.8101, 30.774) -> (-23.4223, 30.774)
  line L108 (-23.4223, 30.774) -> (-23.4223, 30.4628)
  spline S24 degree 2 poles (-22.0712, 30.4085) (-22.4022, 30.4085) (-22.8665, 30.5468) (-23.0716, 30.6456) knots 0 0 0 1 2 2 2
  line L109 (-23.0716, 30.6456) -> (-23.0716, 31.1544)
  line L110 (-23.0716, 31.1544) -> (-23.0419, 31.1544)
  spline S25 degree 2 poles (-23.0419, 31.1544) (-22.8418, 30.9667) (-22.3355, 30.7592) (-22.1008, 30.7592) knots 0 0 0 1 2 2 2
  spline S26 degree 2 poles (-22.1008, 30.7592) (-21.7649, 30.7592) (-21.4216, 31.0383) (-21.4216, 31.268) knots 0 0 0 1 2 2 2
  spline S27 degree 2 poles (-21.4216, 31.268) (-21.4216, 31.4508) (-21.6019, 31.6781) (-21.797, 31.7349) knots 0 0 0 1 2 2 2
  spline S28 degree 2 poles (-21.797, 31.7349) (-21.9378, 31.7744) (-22.1725, 31.8287) (-22.3478, 31.8732) knots 0 0 0 1 2 2 2
  spline S29 degree 2 poles (-22.3478, 31.8732) (-22.5059, 31.9152) (-22.7554, 32.0411) (-22.8517, 32.1424) knots 0 0 0 1 2 2 2
  spline S30 degree 2 poles (-22.8517, 32.1424) (-22.9456, 32.2437) (-23.0493, 32.5154) (-23.0493, 32.6932) knots 0 0 0 1 2 2 2
  spline S31 degree 2 poles (-23.0493, 32.6932) (-23.0493, 33.0637) (-22.4713, 33.5651) (-22.0243, 33.5651) knots 0 0 0 1 2 2 2
  spline S32 degree 2 poles (-22.0243, 33.5651) (-21.7674, 33.5651) (-21.3129, 33.4639) (-21.1178, 33.3675) knots 0 0 0 1 2 2 2
  line L111 (-21.1178, 33.3675) -> (-21.1178, 32.8834)
  line L112 (-21.1178, 32.8834) -> (-21.1474, 32.8834)
  spline S33 degree 2 poles (-21.1474, 32.8834) (-21.2931, 33.0168) (-21.7476, 33.2144) (-21.9971, 33.2144) knots 0 0 0 1 2 2 2
  spline S34 degree 2 poles (-21.9971, 33.2144) (-22.2787, 33.2144) (-22.627, 32.9501) (-22.627, 32.7352) knots 0 0 0 1 2 2 2
  spline S35 degree 2 poles (-22.627, 32.7352) (-22.627, 32.5426) (-22.4219, 32.3128) (-22.2293, 32.261) knots 0 0 0 1 2 2 2
  spline S36 degree 2 poles (-22.2293, 32.261) (-22.1008, 32.2264) (-21.7279, 32.1375) (-21.6044, 32.1004) knots 0 0 0 1 2 2 2
  spline S37 degree 2 poles (-21.6044, 32.1004) (-21.2907, 32.0041) (-20.9992, 31.6163) (-20.9992, 31.3323) knots 0 0 0 1 2 2 2
  spline S38 degree 2 poles (-20.9992, 31.3323) (-20.9992, 31.1519) (-21.1449, 30.8061) (-21.2759, 30.6851) knots 0 0 0 1 2 2 2
  spline S39 degree 2 poles (-21.2759, 30.6851) (-21.4216, 30.5517) (-21.7921, 30.4085) (-22.0712, 30.4085) knots 0 0 0 1 2 2 2
  line L113 (-19.8754, 30.4628) -> (-19.8754, 33.1502)
  line L114 (-19.8754, 33.1502) -> (-20.8979, 33.1502)
  line L115 (-20.8979, 33.1502) -> (-20.8979, 33.5108)
  line L116 (-20.8979, 33.5108) -> (-18.4477, 33.5108)
  line L117 (-18.4477, 33.5108) -> (-18.4477, 33.1502)
  line L118 (-18.4477, 33.1502) -> (-19.4703, 33.1502)
  line L119 (-19.4703, 33.1502) -> (-19.4703, 30.4628)
  line L120 (-19.4703, 30.4628) -> (-19.8754, 30.4628)
  spline S40 degree 2 poles (83.3555, 30.4464) (83.0245, 30.4464) (82.5602, 30.5847) (82.3551, 30.6835) knots 0 0 0 1 2 2 2
  line L121 (82.3551, 30.6835) -> (82.3551, 31.1924)
  line L122 (82.3551, 31.1924) -> (82.3848, 31.1924)
  spline S41 degree 2 poles (82.3848, 31.1924) (82.5849, 31.0046) (83.0912, 30.7972) (83.3259, 30.7972) knots 0 0 0 1 2 2 2
  spline S42 degree 2 poles (83.3259, 30.7972) (83.6618, 30.7972) (84.0051, 31.0763) (84.0051, 31.306) knots 0 0 0 1 2 2 2
  spline S43 degree 2 poles (84.0051, 31.306) (84.0051, 31.4888) (83.8248, 31.716) (83.6297, 31.7728) knots 0 0 0 1 2 2 2
  spline S44 degree 2 poles (83.6297, 31.7728) (83.4889, 31.8123) (83.2542, 31.8667) (83.0789, 31.9111) knots 0 0 0 1 2 2 2
  spline S45 degree 2 poles (83.0789, 31.9111) (82.9208, 31.9531) (82.6713, 32.0791) (82.575, 32.1804) knots 0 0 0 1 2 2 2
  spline S46 degree 2 poles (82.575, 32.1804) (82.4811, 32.2816) (82.3774, 32.5533) (82.3774, 32.7312) knots 0 0 0 1 2 2 2
  spline S47 degree 2 poles (82.3774, 32.7312) (82.3774, 33.1017) (82.9554, 33.6031) (83.4024, 33.6031) knots 0 0 0 1 2 2 2
  spline S48 degree 2 poles (83.4024, 33.6031) (83.6593, 33.6031) (84.1138, 33.5018) (84.3089, 33.4055) knots 0 0 0 1 2 2 2
  line L123 (84.3089, 33.4055) -> (84.3089, 32.9214)
  line L124 (84.3089, 32.9214) -> (84.2793, 32.9214)
  spline S49 degree 2 poles (84.2793, 32.9214) (84.1336, 33.0548) (83.6791, 33.2524) (83.4296, 33.2524) knots 0 0 0 1 2 2 2
  spline S50 degree 2 poles (83.4296, 33.2524) (83.148, 33.2524) (82.7997, 32.9881) (82.7997, 32.7732) knots 0 0 0 1 2 2 2
  spline S51 degree 2 poles (82.7997, 32.7732) (82.7997, 32.5805) (83.0048, 32.3508) (83.1974, 32.2989) knots 0 0 0 1 2 2 2
  spline S52 degree 2 poles (83.1974, 32.2989) (83.3259, 32.2643) (83.6988, 32.1754) (83.8223, 32.1384) knots 0 0 0 1 2 2 2
  spline S53 degree 2 poles (83.8223, 32.1384) (84.136, 32.042) (84.4275, 31.6543) (84.4275, 31.3702) knots 0 0 0 1 2 2 2
  spline S54 degree 2 poles (84.4275, 31.3702) (84.4275, 31.1899) (84.2818, 30.8441) (84.1508, 30.7231) knots 0 0 0 1 2 2 2
  spline S55 degree 2 poles (84.1508, 30.7231) (84.0051, 30.5897) (83.6346, 30.4464) (83.3555, 30.4464) knots 0 0 0 1 2 2 2
  line L125 (85.5513, 30.5008) -> (85.5513, 33.1881)
  line L126 (85.5513, 33.1881) -> (84.5288, 33.1881)
  line L127 (84.5288, 33.1881) -> (84.5288, 33.5488)
  line L128 (84.5288, 33.5488) -> (86.979, 33.5488)
  line L129 (86.979, 33.5488) -> (86.979, 33.1881)
  line L130 (86.979, 33.1881) -> (85.9564, 33.1881)
  line L131 (85.9564, 33.1881) -> (85.9564, 30.5008)
  line L132 (85.9564, 30.5008) -> (85.5513, 30.5008)
  line L133 (88.3499, 30.5008) -> (87.1692, 30.5008)
  line L134 (87.1692, 30.5008) -> (87.1692, 30.812)
  line L135 (87.1692, 30.812) -> (87.557, 30.812)
  line L136 (87.557, 30.812) -> (87.557, 33.2375)
  line L137 (87.557, 33.2375) -> (87.1692, 33.2375)
  line L138 (87.1692, 33.2375) -> (87.1692, 33.5488)
  line L139 (87.1692, 33.5488) -> (88.3499, 33.5488)
  line L140 (88.3499, 33.5488) -> (88.3499, 33.2375)
  line L141 (88.3499, 33.2375) -> (87.9621, 33.2375)
  line L142 (87.9621, 33.2375) -> (87.9621, 30.812)
  line L143 (87.9621, 30.812) -> (88.3499, 30.812)
  line L144 (88.3499, 30.812) -> (88.3499, 30.5008)
  spline S56 degree 2 poles (90.0418, 30.4464) (89.7454, 30.4464) (89.244, 30.6465) (89.0612, 30.8466) knots 0 0 0 1 2 2 2
  spline S57 degree 2 poles (89.0612, 30.8466) (88.8785, 31.0442) (88.6784, 31.637) (88.6784, 32.0223) knots 0 0 0 1 2 2 2
  spline S58 degree 2 poles (88.6784, 32.0223) (88.6784, 32.4051) (88.8735, 32.9732) (89.0588, 33.1832) knots 0 0 0 1 2 2 2
  spline S59 degree 2 poles (89.0588, 33.1832) (89.2416, 33.3882) (89.7405, 33.6031) (90.0492, 33.6031) knots 0 0 0 1 2 2 2
  spline S60 degree 2 poles (90.0492, 33.6031) (90.2024, 33.6031) (90.4716, 33.5586) (90.5852, 33.5241) knots 0 0 0 1 2 2 2
  spline S61 degree 2 poles (90.5852, 33.5241) (90.684, 33.4919) (90.8891, 33.4006) (90.9903, 33.3462) knots 0 0 0 1 2 2 2
  line L145 (90.9903, 33.3462) -> (90.9903, 32.8572)
  line L146 (90.9903, 32.8572) -> (90.9582, 32.8572)
  spline S62 degree 2 poles (90.9582, 32.8572) (90.9039, 32.9066) (90.7359, 33.0449) (90.6149, 33.1116) knots 0 0 0 1 2 2 2
  spline S63 degree 2 poles (90.6149, 33.1116) (90.4988, 33.1758) (90.2246, 33.2573) (90.0468, 33.2573) knots 0 0 0 1 2 2 2
  spline S64 degree 2 poles (90.0468, 33.2573) (89.8516, 33.2573) (89.5034, 33.0967) (89.3725, 32.9436) knots 0 0 0 1 2 2 2
  spline S65 degree 2 poles (89.3725, 32.9436) (89.244, 32.788) (89.1008, 32.3162) (89.1008, 32.0223) knots 0 0 0 1 2 2 2
  spline S66 degree 2 poles (89.1008, 32.0223) (89.1008, 31.7086) (89.2514, 31.2566) (89.3823, 31.101) knots 0 0 0 1 2 2 2
  spline S67 degree 2 poles (89.3823, 31.101) (89.5108, 30.9503) (89.8541, 30.7972) (90.0468, 30.7972) knots 0 0 0 1 2 2 2
  spline S68 degree 2 poles (90.0468, 30.7972) (90.2221, 30.7972) (90.521, 30.8836) (90.6371, 30.9478) knots 0 0 0 1 2 2 2
  spline S69 degree 2 poles (90.6371, 30.9478) (90.7483, 31.0121) (90.9138, 31.1454) (90.9607, 31.1924) knots 0 0 0 1 2 2 2
  line L147 (90.9607, 31.1924) -> (90.9903, 31.1924)
  line L148 (90.9903, 31.1924) -> (90.9903, 30.7082)
  spline S70 degree 2 poles (90.9903, 30.7082) (90.8891, 30.6613) (90.7112, 30.5749) (90.5852, 30.5353) knots 0 0 0 1 2 2 2
  spline S71 degree 2 poles (90.5852, 30.5353) (90.4519, 30.4909) (90.2246, 30.4464) (90.0418, 30.4464) knots 0 0 0 1 2 2 2
  line L149 (93.5913, 30.5008) -> (93.0651, 30.5008)
  line L150 (93.0651, 30.5008) -> (91.9512, 31.9185)
  line L151 (91.9512, 31.9185) -> (91.7733, 31.7185)
  line L152 (91.7733, 31.7185) -> (91.7733, 30.5008)
  line L153 (91.7733, 30.5008) -> (91.3682, 30.5008)
  line L154 (91.3682, 30.5008) -> (91.3682, 33.5488)
  line L155 (91.3682, 33.5488) -> (91.7733, 33.5488)
  line L156 (91.7733, 33.5488) -> (91.7733, 32.1483)
  line L157 (91.7733, 32.1483) -> (93.0231, 33.5488)
  line L158 (93.0231, 33.5488) -> (93.5171, 33.5488)
  line L159 (93.5171, 33.5488) -> (92.255, 32.1878)
  line L160 (92.255, 32.1878) -> (93.5913, 30.5008)
  line L161 (116.5454, 30.5595) -> (116.0193, 30.5595)
  line L162 (116.0193, 30.5595) -> (115.056, 31.7723)
  line L163 (115.056, 31.7723) -> (114.5916, 31.7723)
  line L164 (114.5916, 31.7723) -> (114.5916, 30.5595)
  line L165 (114.5916, 30.5595) -> (114.1866, 30.5595)
  line L166 (114.1866, 30.5595) -> (114.1866, 33.6075)
  line L167 (114.1866, 33.6075) -> (114.972, 33.6075)
  spline S72 degree 2 poles (114.972, 33.6075) (115.2338, 33.6075) (115.5871, 33.5507) (115.7476, 33.4469) knots 0 0 0 1 2 2 2
  spline S73 degree 2 poles (115.7476, 33.4469) (115.9082, 33.3432) (116.0934, 33.0196) (116.0934, 32.78) knots 0 0 0 1 2 2 2
  spline S74 degree 2 poles (116.0934, 32.78) (116.0934, 32.4466) (115.7526, 31.9946) (115.4611, 31.8859) knots 0 0 0 1 2 2 2
  line L168 (115.4611, 31.8859) -> (116.5454, 30.5595)
  spline S75 degree 2 poles (115.671, 32.7479) (115.671, 32.8813) (115.5772, 33.0863) (115.4784, 33.153) knots 0 0 0 1 2 2 2
  spline S76 degree 2 poles (115.4784, 33.153) (115.3919, 33.2098) (115.1622, 33.2567) (114.9943, 33.2567) knots 0 0 0 1 2 2 2
  line L169 (114.9943, 33.2567) -> (114.5916, 33.2567)
  line L170 (114.5916, 33.2567) -> (114.5916, 32.1106)
  line L171 (114.5916, 32.1106) -> (114.9473, 32.1106)
  spline S77 degree 2 poles (114.9473, 32.1106) (115.1227, 32.1106) (115.4018, 32.1724) (115.4981, 32.2687) knots 0 0 0 1 2 2 2
  spline S78 degree 2 poles (115.4981, 32.2687) (115.5871, 32.3527) (115.671, 32.5898) (115.671, 32.7479) knots 0 0 0 1 2 2 2
  line L172 (116.7875, 30.5595) -> (116.7875, 33.6075)
  line L173 (116.7875, 33.6075) -> (118.6943, 33.6075)
  line L174 (118.6943, 33.6075) -> (118.6943, 33.2469)
  line L175 (118.6943, 33.2469) -> (117.1926, 33.2469)
  line L176 (117.1926, 33.2469) -> (117.1926, 32.412)
  line L177 (117.1926, 32.412) -> (118.5931, 32.412)
  line L178 (118.5931, 32.412) -> (118.5931, 32.0514)
  line L179 (118.5931, 32.0514) -> (117.1926, 32.0514)
  line L180 (117.1926, 32.0514) -> (117.1926, 30.9201)
  line L181 (117.1926, 30.9201) -> (118.6943, 30.9201)
  line L182 (118.6943, 30.9201) -> (118.6943, 30.5595)
  line L183 (118.6943, 30.5595) -> (116.7875, 30.5595)
  spline S79 degree 2 poles (119.9886, 30.5051) (119.6576, 30.5051) (119.1933, 30.6435) (118.9883, 30.7423) knots 0 0 0 1 2 2 2
  line L184 (118.9883, 30.7423) -> (118.9883, 31.2511)
  line L185 (118.9883, 31.2511) -> (119.0179, 31.2511)
  spline S80 degree 2 poles (119.0179, 31.2511) (119.218, 31.0634) (119.7243, 30.8559) (119.959, 30.8559) knots 0 0 0 1 2 2 2
  spline S81 degree 2 poles (119.959, 30.8559) (120.2949, 30.8559) (120.6382, 31.135) (120.6382, 31.3647) knots 0 0 0 1 2 2 2
  spline S82 degree 2 poles (120.6382, 31.3647) (120.6382, 31.5475) (120.4579, 31.7747) (120.2628, 31.8315) knots 0 0 0 1 2 2 2
  spline S83 degree 2 poles (120.2628, 31.8315) (120.122, 31.8711) (119.8874, 31.9254) (119.712, 31.9699) knots 0 0 0 1 2 2 2
  spline S84 degree 2 poles (119.712, 31.9699) (119.5539, 32.0118) (119.3044, 32.1378) (119.2081, 32.2391) knots 0 0 0 1 2 2 2
  spline S85 degree 2 poles (119.2081, 32.2391) (119.1142, 32.3404) (119.0105, 32.6121) (119.0105, 32.7899) knots 0 0 0 1 2 2 2
  spline S86 degree 2 poles (119.0105, 32.7899) (119.0105, 33.1604) (119.5885, 33.6618) (120.0356, 33.6618) knots 0 0 0 1 2 2 2
  spline S87 degree 2 poles (120.0356, 33.6618) (120.2924, 33.6618) (120.7469, 33.5605) (120.9421, 33.4642) knots 0 0 0 1 2 2 2
  line L186 (120.9421, 33.4642) -> (120.9421, 32.9801)
  line L187 (120.9421, 32.9801) -> (120.9124, 32.9801)
  spline S88 degree 2 poles (120.9124, 32.9801) (120.7667, 33.1135) (120.3122, 33.3111) (120.0627, 33.3111) knots 0 0 0 1 2 2 2
  spline S89 degree 2 poles (120.0627, 33.3111) (119.7811, 33.3111) (119.4329, 33.0468) (119.4329, 32.8319) knots 0 0 0 1 2 2 2
  spline S90 degree 2 poles (119.4329, 32.8319) (119.4329, 32.6392) (119.6379, 32.4095) (119.8306, 32.3576) knots 0 0 0 1 2 2 2
  spline S91 degree 2 poles (119.8306, 32.3576) (119.959, 32.3231) (120.332, 32.2341) (120.4555, 32.1971) knots 0 0 0 1 2 2 2
  spline S92 degree 2 poles (120.4555, 32.1971) (120.7692, 32.1008) (121.0606, 31.713) (121.0606, 31.4289) knots 0 0 0 1 2 2 2
  spline S93 degree 2 poles (121.0606, 31.4289) (121.0606, 31.2486) (120.9149, 30.9028) (120.784, 30.7818) knots 0 0 0 1 2 2 2
  spline S94 degree 2 poles (120.784, 30.7818) (120.6382, 30.6484) (120.2677, 30.5051) (119.9886, 30.5051) knots 0 0 0 1 2 2 2
  line L188 (121.4731, 30.5595) -> (121.4731, 33.6075)
  line L189 (121.4731, 33.6075) -> (123.38, 33.6075)
  line L190 (123.38, 33.6075) -> (123.38, 33.2469)
  line L191 (123.38, 33.2469) -> (121.8782, 33.2469)
  line L192 (121.8782, 33.2469) -> (121.8782, 32.412)
  line L193 (121.8782, 32.412) -> (123.2787, 32.412)
  line L194 (123.2787, 32.412) -> (123.2787, 32.0514)
  line L195 (123.2787, 32.0514) -> (121.8782, 32.0514)
  line L196 (121.8782, 32.0514) -> (121.8782, 30.9201)
  line L197 (121.8782, 30.9201) -> (123.38, 30.9201)
  line L198 (123.38, 30.9201) -> (123.38, 30.5595)
  line L199 (123.38, 30.5595) -> (121.4731, 30.5595)
  line L200 (124.5359, 30.5595) -> (124.5359, 33.2469)
  line L201 (124.5359, 33.2469) -> (123.5133, 33.2469)
  line L202 (123.5133, 33.2469) -> (123.5133, 33.6075)
  line L203 (123.5133, 33.6075) -> (125.9636, 33.6075)
  line L204 (125.9636, 33.6075) -> (125.9636, 33.2469)
  line L205 (125.9636, 33.2469) -> (124.941, 33.2469)
  line L206 (124.941, 33.2469) -> (124.941, 30.5595)
  line L207 (124.941, 30.5595) -> (124.5359, 30.5595)
  point P0 (66, -5.1)
  constraints: 8 other
extrude "Extrusion35" add sketch "Sketch46" along normal blind 1
body "Solid1"
